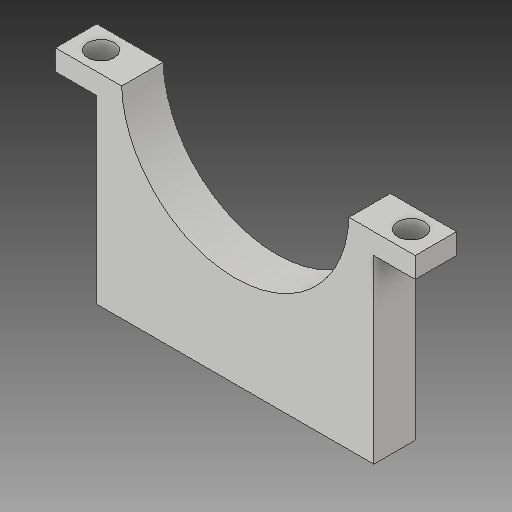
# Autodesk Inventor part: REAL MOTOR MOUNT 2.75 TOP
Saved by Autodesk Inventor 2019 (Build 230136000, 136)
## iProperties
Created: 2018-01-16
Part Number: REAL MOTOR MOUNT 2.75 TOP
Material: Generic
Document SubType Name: Modeling
Designer: Administrator
Density: 1 g/cm^3
Appearance: Default
Author: Administrator
Autodesk Inventor part; units mm, degrees
ref_plane "YZ Plane" through (0, 0, 0) normal (1, 0, 0) x (0, 1, 0)
ref_plane "XZ Plane" through (0, 0, 0) normal (0, 1, 0) x (-1, 0, 0)
ref_plane "XY Plane" through (0, 0, 0) normal (0, 0, 1) x (1, 0, 0)
sketch "Sketch1" plane through (0, 0, 0) normal (0, 0, 1) x (1, 0, 0)
  line L0 (-39.344, -1.4316) -> (-39.3671, -1.4316)
  line L1 (-39.344, -1.4316) -> (-52.044, -1.4316)
  line L2 (-39.344, -1.4316) -> (-45.694, -1.4316)
  line L3 (-39.344, -1.4316) -> (-46.964, -1.4316)
  line L4 (-46.964, -1.4316) -> (-46.964, -22.4724)
  line L5 (-46.964, -7.7816) -> (-59.664, -7.7816)
  line L6 (-59.664, -7.7816) -> (-59.664, -1.4316)
  arc A0 (-39.344, -1.4316) -> (30.4598, -1.4316) centre (-4.4421, -0.1616) ccw
  line L7 (30.4598, -1.4316) -> (43.1598, -1.4316)
  arc A1 (-46.964, -22.4724) -> (38.0798, -22.4724) centre (-4.4421, -0.1616) ccw
  line L8 (30.4598, -1.4316) -> (38.0798, -1.4316)
  line L9 (38.0798, -1.4316) -> (38.0798, -22.4724)
  line L10 (38.0798, -7.7816) -> (50.7798, -7.7816)
  line L11 (50.7798, -7.7816) -> (50.7798, -1.4316)
  line L12 (43.1598, -1.4316) -> (50.7798, -1.4316)
  line L13 (-52.044, -1.4316) -> (-59.664, -1.4316)
  line L14 (-46.964, -42.5386) -> (-46.964, -22.4724)
  line L15 (-46.964, -63.265) -> (-46.964, -42.5386)
  line L16 (-46.964, -22.4724) -> (-31.3118, -22.4724)
  line L17 (24.2345, -20.0969) -> (38.1472, -20.0969)
  line L18 (38.0798, -22.4724) -> (38.0798, -63.265)
  line L19 (38.0798, -63.265) -> (-46.964, -63.265)
  point P0 (0, 0)
  point P1 (0, 0)
  dimension "d0" = 69.85
  dimension "d1" = 12.7
  dimension "d2" = 12.7
  dimension "d3" = 7.62
  dimension "d4" = 7.62
  dimension "d5" = 7.62
  dimension "d6" = 7.62
  dimension "d7" = 6.35
  dimension "d8" = 6.35
  dimension "d17" = 61.8334
  constraints: 40 end point, 7 horizontal, 6 point on circle, 5 point on line, 3 perpendicular, 3 vertical, 2 centre point, 1 coincident, 1 concentric, 1 midpoint
  measures "d0" diameter of A0
  measures "d1" distance of L8.start L7.end
  measures "d2" distance of L0.start L1.end
  measures "d3" distance of L1.end L6.end
  measures "d4" distance of L7.end L11.end
  measures "d5" distance of L8.start L9.start
  measures "d6" distance of L0.start L3.end
  measures "d7" distance of L5.end L6.end
  measures "d8" distance of L11.start L11.end
  measures "d17" distance between parallel lines of L8 L19
extrude "Extrusion1" add sketch "Sketch1" along normal blind 12.7
sketch "Sketch2" plane through (-59.664, -1.4316, 0) normal (0, 1, 0) x (1, 0, 0)
  circle A0 centre (7.62, -6.35) radius 4.064
  circle A1 centre (102.8238, -6.35) radius 4.064
  line L0 (90.1238, 0) -> (90.1238, -12.7) projected
  line L1 (20.32, 0) -> (20.32, -12.7) projected
  point P0 (59.664, 0)
  dimension "d11" = 12.7
  dimension "d12" = 12.7
  dimension "d13" = 8.128
  dimension "d14" = 8.128
  constraints: 2 centre point
  measures "d11" distance from line of L0 A1.centre
  measures "d12" distance from line of L1 A0.centre
  measures "d13" diameter of A0
  measures "d14" diameter of A1
extrude "Extrusion2" cut sketch "Sketch2" against normal blind 25.4
body "Solid1"
